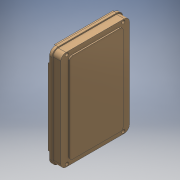
# Autodesk Inventor part: ET6
Saved by Autodesk Inventor 2016 (Build 200138000, 138)
## iProperties
Created: 2016-03-20
Part Number: ET6
Material: Genérico
Document SubType Name: Modeling
Designer: Usuario1
Density: 1 g/cm^3
Appearance: Valor por defecto
Author: Usuario1
Autodesk Inventor part; units mm, degrees
ref_plane "YZ Plane" through (0, 0, 0) normal (1, 0, 0) x (0, 1, 0)
ref_plane "XZ Plane" through (0, 0, 0) normal (0, 1, 0) x (-1, 0, 0)
ref_plane "XY Plane" through (0, 0, 0) normal (0, 0, 1) x (1, 0, 0)
sketch "Boceto1" plane through (0, 0, 0) normal (1, 0, 0) x (0, 1, 0)
  circle A0 centre (0.279944, 0.10542) radius 0.062268
  circle A1 centre (2.482962, 0.10542) radius 0.062268
  circle A2 centre (2.482962, -3.59176) radius 0.062268
  line L0 (0.335673, -3.37176) -> (0.335673, -0.11458)
  arc A3 (0.335673, -3.37176) -> (0.455673, -3.49176) centre (0.455673, -3.37176) ccw
  line L1 (0.455673, 0.00542) -> (2.307232, 0.00542)
  arc A4 (0.455673, 0.00542) -> (0.335673, -0.11458) centre (0.455673, -0.11458) ccw
  arc A5 (2.427232, -0.11458) -> (2.307232, 0.00542) centre (2.307232, -0.11458) ccw
  line L2 (2.427232, -0.11458) -> (2.427232, -3.37176)
  arc A6 (2.307232, -3.49176) -> (2.427232, -3.37176) centre (2.307232, -3.37176) ccw
  line L3 (2.307232, -3.49176) -> (0.455673, -3.49176)
  line L4 (0, -3.48634) -> (0, 0)
  arc A7 (0.24, 0.24) -> (0, 0) centre (0.24, 0) ccw
  line L5 (0.24, 0.24) -> (2.522906, 0.24)
  arc A8 (2.762906, 0) -> (2.522906, 0.24) centre (2.522906, 0) ccw
  line L6 (2.762906, 0) -> (2.762906, -3.48634)
  arc A9 (2.522906, -3.72634) -> (2.762906, -3.48634) centre (2.522906, -3.48634) ccw
  line L7 (2.522906, -3.72634) -> (0.24, -3.72634)
  arc A10 (0, -3.48634) -> (0.24, -3.72634) centre (0.24, -3.48634) ccw
  line L8 (2.718635, -3.48207) -> (2.718635, -0.004271)
  arc A11 (2.718635, -0.004271) -> (2.518635, 0.195729) centre (2.518635, -0.004271) ccw
  line L9 (2.518635, 0.195729) -> (0.244271, 0.195729)
  arc A12 (0.244271, 0.195729) -> (0.044271, -0.004271) centre (0.244271, -0.004271) ccw
  line L10 (0.044271, -0.004271) -> (0.044271, -3.48207)
  arc A13 (0.044271, -3.48207) -> (0.244271, -3.68207) centre (0.244271, -3.48207) ccw
  line L11 (0.244271, -3.68207) -> (2.518635, -3.68207)
  arc A14 (2.518635, -3.68207) -> (2.718635, -3.48207) centre (2.518635, -3.48207) ccw
  circle A15 centre (0.279944, -3.59176) radius 0.062268
  constraints: 24 end point, 24 point on circle, 16 centre point
extrude "Extrusión1" add sketch "Boceto1" along normal blind 0.15 contours L0 A4 L1 A5 L2 A6 L3 A3 | L4 A7 L5 A8 L6 A9 L7 A10 | A14 L11 A13 L10 A12 L9 A11 L8
sketch "Boceto2" plane through (0.15, 0, 0) normal (1, 0, 0) x (0, 0, -1)
  circle A0 centre (3.59176, 2.482962) radius 0.062268
  circle A1 centre (3.59176, 0.279944) radius 0.062268
  circle A2 centre (-0.10542, 0.279944) radius 0.062268
  line L0 (0.11458, 2.427232) -> (3.37176, 2.427232)
  arc A3 (0.11458, 2.427232) -> (-0.00542, 2.307232) centre (0.11458, 2.307232) ccw
  line L1 (3.49176, 2.307232) -> (3.49176, 0.455673)
  arc A4 (3.49176, 2.307232) -> (3.37176, 2.427232) centre (3.37176, 2.307232) ccw
  arc A5 (3.37176, 0.335673) -> (3.49176, 0.455673) centre (3.37176, 0.455673) ccw
  line L2 (3.37176, 0.335673) -> (0.11458, 0.335673)
  arc A6 (-0.00542, 0.455673) -> (0.11458, 0.335673) centre (0.11458, 0.455673) ccw
  line L3 (-0.00542, 0.455673) -> (-0.00542, 2.307232)
  line L4 (0, 2.762906) -> (3.48634, 2.762906)
  arc A7 (3.72634, 2.522906) -> (3.48634, 2.762906) centre (3.48634, 2.522906) ccw
  line L5 (3.72634, 2.522906) -> (3.72634, 0.24)
  arc A8 (3.48634, 0) -> (3.72634, 0.24) centre (3.48634, 0.24) ccw
  line L6 (3.48634, 0) -> (0, 0)
  arc A9 (-0.24, 0.24) -> (0, 0) centre (0, 0.24) ccw
  line L7 (-0.24, 0.24) -> (-0.24, 2.522906)
  arc A10 (0, 2.762906) -> (-0.24, 2.522906) centre (0, 2.522906) ccw
  line L8 (0.004271, 0.044271) -> (3.48207, 0.044271)
  arc A11 (3.48207, 0.044271) -> (3.68207, 0.244271) centre (3.48207, 0.244271) ccw
  line L9 (3.68207, 0.244271) -> (3.68207, 2.518635)
  arc A12 (3.68207, 2.518635) -> (3.48207, 2.718635) centre (3.48207, 2.518635) ccw
  line L10 (3.48207, 2.718635) -> (0.004271, 2.718635)
  arc A13 (0.004271, 2.718635) -> (-0.195729, 2.518635) centre (0.004271, 2.518635) ccw
  line L11 (-0.195729, 2.518635) -> (-0.195729, 0.244271)
  arc A14 (-0.195729, 0.244271) -> (0.004271, 0.044271) centre (0.004271, 0.244271) ccw
  circle A15 centre (-0.10542, 2.482962) radius 0.062268
  circle A16 centre (3.59176, 0.279944) radius 0.062268
  circle A17 centre (3.59176, 2.482962) radius 0.062268
  circle A18 centre (-0.10542, 2.482962) radius 0.062268
  circle A19 centre (-0.10542, 0.279944) radius 0.062268
  line L12 (0, 0) -> (3.48634, 0)
  arc A20 (3.48634, 0) -> (3.72634, 0.24) centre (3.48634, 0.24) ccw
  line L13 (3.72634, 0.24) -> (3.72634, 2.522906)
  arc A21 (3.72634, 2.522906) -> (3.48634, 2.762906) centre (3.48634, 2.522906) ccw
  line L14 (3.48634, 2.762906) -> (0, 2.762906)
  arc A22 (0, 2.762906) -> (-0.24, 2.522906) centre (0, 2.522906) ccw
  line L15 (-0.24, 2.522906) -> (-0.24, 0.24)
  arc A23 (-0.24, 0.24) -> (0, 0) centre (0, 0.24) ccw
  constraints: 24 end point, 24 point on circle, 16 centre point
extrude "Extrusión2" add sketch "Boceto2" along normal blind 0.3 contours L0 A4 L1 A5 L2 A6 L3 A3 | A14 L11 A13 L10 A12 L9 A11 L8
sketch "Boceto3" plane through (0.45, 0, 0) normal (1, 0, 0) x (0, 0, -1)
  circle A0 centre (-0.10542, 2.482962) radius 0.062268
  circle A1 centre (-0.10542, 0.279944) radius 0.062268
  circle A2 centre (3.59176, 0.279944) radius 0.062268
  circle A3 centre (3.59176, 2.482962) radius 0.062268
  line L0 (0.004271, 0.044271) -> (3.48207, 0.044271)
  arc A4 (3.48207, 0.044271) -> (3.68207, 0.244271) centre (3.48207, 0.244271) ccw
  line L1 (3.68207, 0.244271) -> (3.68207, 2.518635)
  arc A5 (3.68207, 2.518635) -> (3.48207, 2.718635) centre (3.48207, 2.518635) ccw
  line L2 (3.48207, 2.718635) -> (0.004271, 2.718635)
  arc A6 (0.004271, 2.718635) -> (-0.195729, 2.518635) centre (0.004271, 2.518635) ccw
  line L3 (-0.195729, 2.518635) -> (-0.195729, 0.244271)
  arc A7 (-0.195729, 0.244271) -> (0.004271, 0.044271) centre (0.004271, 0.244271) ccw
  circle A8 centre (3.59176, 2.482962) radius 0.062268
  circle A9 centre (3.59176, 0.279944) radius 0.062268
  circle A10 centre (-0.10542, 0.279944) radius 0.062268
  line L4 (0.11458, 2.427232) -> (3.37176, 2.427232)
  arc A11 (0.11458, 2.427232) -> (-0.00542, 2.307232) centre (0.11458, 2.307232) ccw
  line L5 (3.49176, 2.307232) -> (3.49176, 0.455673)
  arc A12 (3.49176, 2.307232) -> (3.37176, 2.427232) centre (3.37176, 2.307232) ccw
  arc A13 (3.37176, 0.335673) -> (3.49176, 0.455673) centre (3.37176, 0.455673) ccw
  line L6 (3.37176, 0.335673) -> (0.11458, 0.335673)
  arc A14 (-0.00542, 0.455673) -> (0.11458, 0.335673) centre (0.11458, 0.455673) ccw
  line L7 (-0.00542, 0.455673) -> (-0.00542, 2.307232)
  line L8 (0, 2.762906) -> (3.48634, 2.762906)
  arc A15 (3.72634, 2.522906) -> (3.48634, 2.762906) centre (3.48634, 2.522906) ccw
  line L9 (3.72634, 2.522906) -> (3.72634, 0.24)
  arc A16 (3.48634, 0) -> (3.72634, 0.24) centre (3.48634, 0.24) ccw
  line L10 (3.48634, 0) -> (0, 0)
  arc A17 (-0.24, 0.24) -> (0, 0) centre (0, 0.24) ccw
  line L11 (-0.24, 0.24) -> (-0.24, 2.522906)
  arc A18 (0, 2.762906) -> (-0.24, 2.522906) centre (0, 2.522906) ccw
  line L12 (0.004271, 0.044271) -> (3.48207, 0.044271)
  arc A19 (3.48207, 0.044271) -> (3.68207, 0.244271) centre (3.48207, 0.244271) ccw
  line L13 (3.68207, 0.244271) -> (3.68207, 2.518635)
  arc A20 (3.68207, 2.518635) -> (3.48207, 2.718635) centre (3.48207, 2.518635) ccw
  line L14 (3.48207, 2.718635) -> (0.004271, 2.718635)
  arc A21 (0.004271, 2.718635) -> (-0.195729, 2.518635) centre (0.004271, 2.518635) ccw
  line L15 (-0.195729, 2.518635) -> (-0.195729, 0.244271)
  arc A22 (-0.195729, 0.244271) -> (0.004271, 0.044271) centre (0.004271, 0.244271) ccw
  circle A23 centre (-0.10542, 2.482962) radius 0.062268
  point P0 (0, 0)
  constraints: 24 end point, 24 point on circle, 16 centre point
extrude "Extrusión3" add sketch "Boceto3" along normal blind 0.05 contours L4 A12 L5 A13 L6 A14 L7 A11
sketch "Boceto4" plane through (0, 0, 0) normal (-1, 0, 0) x (0, 0, 1)
  line L0 (0.23996, 0) -> (0.23996, 2.762906)
  line L1 (0.23996, 2.762906) -> (-0.26004, 2.762906)
  line L2 (-0.26004, 2.100874) -> (-0.26004, 2.762906)
  line L3 (0.08996, 2.100874) -> (-0.26004, 2.100874)
  line L4 (0.08996, 0.832183) -> (0.08996, 2.100874)
  line L5 (0.08996, 0.832183) -> (-0.26004, 0.832183)
  line L6 (-0.26004, 0) -> (-0.26004, 0.832183)
  line L7 (0.08996, 0) -> (-0.26004, 0)
  line L8 (0.23996, 0) -> (0.08996, 0)
  line L9 (-3.72634, 0) -> (-3.72634, 2.762906)
  line L10 (-3.72634, 0) -> (-3.57634, 0)
  line L11 (-3.57634, 0) -> (-3.22634, 0)
  line L12 (-3.22634, 0.832183) -> (-3.22634, 0)
  line L13 (-3.57634, 0.832183) -> (-3.22634, 0.832183)
  line L14 (-3.57634, 2.100874) -> (-3.57634, 0.832183)
  line L15 (-3.57634, 2.100874) -> (-3.22634, 2.100874)
  line L16 (-3.22634, 2.762906) -> (-3.22634, 2.100874)
  line L17 (-3.72634, 2.762906) -> (-3.22634, 2.762906)
  circle A0 centre (-3.59176, 0.279944) radius 0.062268
  circle A1 centre (-3.59176, 2.482962) radius 0.062268
  circle A2 centre (0.10542, 2.482962) radius 0.062268
  circle A3 centre (0.10542, 0.279944) radius 0.062268
  line L18 (-3.48634, 0) -> (0, 0)
  arc A4 (0, 0) -> (0.24, 0.24) centre (0, 0.24) ccw
  line L19 (0.24, 0.24) -> (0.24, 2.522906)
  arc A5 (0.24, 2.522906) -> (0, 2.762906) centre (0, 2.522906) ccw
  line L20 (0, 2.762906) -> (-3.48634, 2.762906)
  arc A6 (-3.48634, 2.762906) -> (-3.72634, 2.522906) centre (-3.48634, 2.522906) ccw
  line L21 (-3.72634, 2.522906) -> (-3.72634, 0.24)
  arc A7 (-3.72634, 0.24) -> (-3.48634, 0) centre (-3.48634, 0.24) ccw
  line L22 (-3.72634, 1.381453) -> (0.24, 1.381453)
  line L23 (0.24, 0.24) -> (0.24, 2.522906)
  point P0 (-3.72634, -0.118538)
  constraints: 38 end point, 2 midpoint
extrude "Extrusión4" cut sketch "Boceto4" against normal blind 0.05 contours L8 L7 A4 L0 | A4 L7 L6 L5 L4 L22 L0 | L22 L4 L3 L2 L1 A5 L0 | A5 L1 L0 | L22 L9 A6 L17 L16 L15 L14 | L14 L13 L12 L11 A7 L9 L22 | L11 L10 L9 A7 | L9 L17 A6
